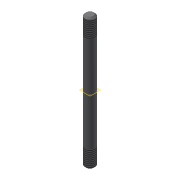
# Autodesk Inventor part: HandleBody
Saved by Autodesk Inventor 2022 Beta2 (Build 260130000, 130) ContinuousBuild 0
## iProperties
Created: 2011-02-11
Part Number: HandleBody
Material: Generic
Document SubType Name: Modeling
Designer: landrews
Density: 1 g/cm^3
Appearance: Light Gray
Author: landrews
Autodesk Inventor part; units mm, degrees
ref_plane "YZ Plane" through (0, 0, 0) normal (1, 0, 0) x (0, 1, 0)
ref_plane "XZ Plane" through (0, 0, 0) normal (0, 1, 0) x (-1, 0, 0)
sketch "Sketch1" plane through (0, 0, 0) normal (0, 0, 1) x (1, 0, 0)
  circle A0 centre (0, 0) radius 3
  dimension "d0" = 6
  constraints: 1 centre point, 1 coincident
  measures "d0" diameter of A0
extrude "Extrusion1" add sketch "Sketch1" along normal mid plane 80
chamfer "Chamfer2" distance 1 angle 45 2 edges at (-3, 0, -40) (-3, 0, 40)
thread "Thread1" size "M6x1" class "6g" standard "ANSI Metric M Profile" length 10
thread "Thread2" size "M6x1" class "6g" standard "ANSI Metric M Profile" length 10
body "Solid1"
